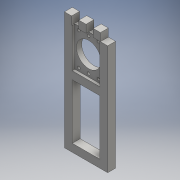
# Autodesk Inventor part: framesideRight
Saved by Autodesk Inventor 2016 (Build 200138000, 138)
## iProperties
Created: 2016-05-18
Part Number: framesideRight
Material: Generic
Document SubType Name: Modeling
Designer: hesaon
Density: 1 g/cm^3
Appearance: Default
Author: hesaon
Autodesk Inventor part; units mm, degrees
ref_plane "YZ Plane" through (0, 0, 0) normal (1, 0, 0) x (0, 1, 0)
ref_plane "XZ Plane" through (0, 0, 0) normal (0, 1, 0) x (-1, 0, 0)
ref_plane "XY Plane" through (0, 0, 0) normal (0, 0, 1) x (1, 0, 0)
sketch "Sketch1" plane through (0, 0, 0) normal (0, 1, 0) x (-1, 0, 0)
  line L0 (0, 0) -> (66, 0)
  line L1 (66, 0) -> (66, -180)
  line L2 (66, -180) -> (0, -180)
  line L3 (0, -180) -> (0, 0)
  line L4 (54, -12) -> (12, -12)
  line L5 (12, -168) -> (54, -168)
  line L6 (54, -72) -> (12, -72)
  line L7 (54, -84) -> (12, -84)
  line L8 (54, -168) -> (54, -84)
  line L9 (54, -72) -> (54, -12)
  line L10 (12, -12) -> (12, -72)
  line L11 (12, -84) -> (12, -168)
  dimension "d0" = 66
  dimension "d1" = 180
  dimension "d3" = 42
  dimension "d4" = 12
  dimension "d5" = 12
  dimension "d6" = 60
  dimension "d7" = 12
  dimension "d8" = 12
  dimension "d9" = 12
  constraints: 24 end point, 7 perpendicular, 6 parallel, 2 horizontal, 1 collinear
  measures "d0" distance of L1.end L2.end
  measures "d1" distance of L0.end L1.end
  measures "d3" distance of L5.start L5.end
  measures "d4" distance from line of L2 L5.start
  measures "d5" distance from line of L1 L5.end
  measures "d6" distance of L4.end L6.end
  measures "d7" distance of L7.end L6.end
  measures "d8" distance between parallel lines of L0 L4
  measures "d9" distance from line of L3 L4.end
extrude "Extrusion1" add sketch "Sketch1" along normal blind 12
sketch "Sketch2" plane through (0, 12, 0) normal (0, 1, 0) x (1, 0, 0)
  circle A0 centre (-48, 17) radius 2.1
  circle A1 centre (-33, 17) radius 2.1
  circle A2 centre (-18, 17) radius 2.1
  circle A3 centre (-48, 67) radius 2.1
  circle A4 centre (-33, 67) radius 2.1
  circle A5 centre (-18, 67) radius 2.1
  line L0 (-12, 12) -> (-12, 72) projected
  line L1 (-12, 12) -> (-54, 12) projected
  line L2 (-12, 72) -> (-54, 72) projected
  line L3 (-54, 12) -> (-12, 12) projected
  line L4 (-54, 12) -> (-54, 72)
  line L5 (-54, 12) -> (-54, 72) projected
  line L6 (-54, 12) -> (-12, 12)
  line L7 (-12, 72) -> (-12, 12) projected
  line L8 (-12, 12) -> (-12, 72)
  line L9 (-12, 72) -> (-54, 72)
  dimension "d12" = 4.2
  dimension "d13" = 4.2
  dimension "d15" = 4.2
  dimension "d16" = 4.2
  dimension "d17" = 4.2
  dimension "d42" = 21
  dimension "d43" = 21
  dimension "d44" = 15
  dimension "d45" = 15
  dimension "d46" = 15
  dimension "d47" = 15
  dimension "d48" = 4.2
  dimension "d49" = 5
  dimension "d50" = 5
  dimension "d51" = 5
  dimension "d52" = 5
  dimension "d53" = 5
  constraints: 8 end point, 6 centre point, 2 perpendicular, 1 collinear, 1 vertical
  measures "d12" diameter of A0
  measures "d13" diameter of A1
  measures "d15" diameter of A3
  measures "d16" diameter of A4
  measures "d17" diameter of A5
  measures "d42" distance from line of L0 A1.centre
  measures "d43" distance from line of L0 A4.centre
  measures "d44" distance of A4.centre A5.centre
  measures "d45" distance of A4.centre A3.centre
  measures "d46" distance of A1.centre A0.centre
  measures "d47" distance of A2.centre A1.centre
  measures "d48" diameter of A2
  measures "d49" distance from line of L1 A1.centre
  measures "d50" distance from line of L2 A4.centre
  measures "d51" distance from line of L2 A5.centre
  measures "d52" distance from line of L2 A3.centre
  measures "d53" distance from line of L1 A0.centre
extrude "Extrusion2" add sketch "Sketch2" against normal blind 8
sketch "Sketch3" plane through (0, 4, 0) normal (0, -1, 0) x (1, 0, 0)
  circle A0 centre (-33, -42) radius 18.75
  line L0 (-12, -12) -> (-12, -72) projected
  line L1 (-12, -72) -> (-54, -72) projected
  point P0 (0, 0)
  dimension "d56" = 37.5
  dimension "d57" = 21
  dimension "d58" = 30
  constraints: 1 centre point
  measures "d56" diameter of A0
  measures "d57" distance from line of L0 A0.centre
  measures "d58" distance from line of L1 A0.centre
extrude "Extrusion3" cut sketch "Sketch3" against normal up to next
sketch "Sketch4" plane through (0, 0, 0) normal (0, -1, 0) x (1, 0, 0)
  line L0 (-66, 0) -> (-66, -180) projected
  line L1 (0, 0) -> (-11, 0)
  line L2 (-11, 0) -> (-11, -12)
  line L3 (-11, -12) -> (0, -12)
  line L4 (0, -12) -> (0, 0)
  line L5 (-11, 0) -> (-22, 0)
  line L6 (-22, 0) -> (-22, -12)
  line L7 (-22, -12) -> (-11, -12)
  line L8 (-11, -12) -> (-11, 0)
  line L9 (-54, -12) -> (-12, -12) projected
  line L10 (-22, 0) -> (-33, 0)
  line L11 (-33, 0) -> (-33, -12)
  line L12 (-33, -12) -> (-22, -12)
  line L13 (-22, -12) -> (-22, 0)
  line L14 (-33, 0) -> (-44, 0)
  line L15 (-44, 0) -> (-44, -12)
  line L16 (-44, -12) -> (-33, -12)
  line L17 (-33, -12) -> (-33, 0)
  line L18 (-44, 0) -> (-55, 0)
  line L19 (-55, 0) -> (-55, -12)
  line L20 (-55, -12) -> (-44, -12)
  line L21 (-44, -12) -> (-44, 0)
  line L22 (-55, 0) -> (-66, 0)
  line L23 (-66, 0) -> (-66, -12)
  line L24 (-66, -12) -> (-55, -12)
  line L25 (-55, -12) -> (-55, 0)
  dimension "d79" = 12
  dimension "d80" = 11
  dimension "d81" = 11
  dimension "d82" = 12
  dimension "d83" = 11
  dimension "d84" = 11
  constraints: 48 end point, 12 parallel, 6 horizontal, 6 perpendicular, 4 point on line, 1 coincident, 1 midpoint
  measures "d79" distance of L3.end L1.start
  measures "d80" distance of L2.end L3.end
  measures "d81" distance of L7.end L6.end
  measures "d82" distance of L6.end L5.end
  measures "d83" distance of L16.end L15.end
  measures "d84" distance of L20.end L19.end
extrude "Extrusion4" cut sketch "Sketch4" against normal up to next contours L18 L15 L9 L20 L19 | L10 L6 L9 L11 | L1 L4 L3 L2
body "Solid1"
